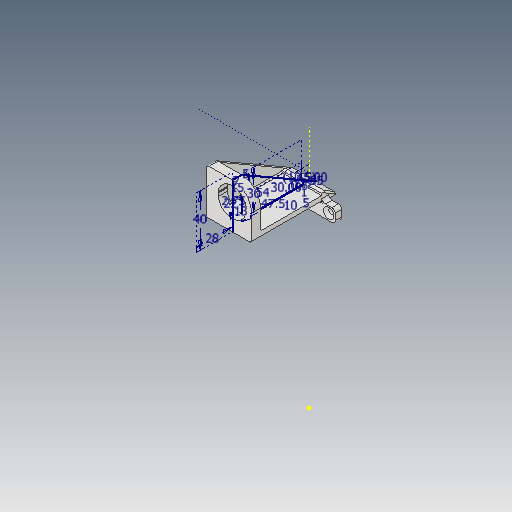
# Autodesk Inventor part: Mount_Killswitch
Saved by Autodesk Inventor 2018.2 (Build 222227000, 227)
## iProperties
Created: 2018-02-23
Part Number: Mount_Killswitch
Material: ABS Plastic
Document SubType Name: Modeling
Designer: NicK Foo
Density: 1.06 g/cm^3
Appearance: Smooth - White
Author: NicK Foo
Autodesk Inventor part; units mm, degrees
ref_plane "YZ Plane" through (0, 0, 0) normal (1, 0, 0) x (0, 1, 0)
ref_plane "XZ Plane" through (0, 0, 0) normal (0, 1, 0) x (-1, 0, 0)
ref_plane "XY Plane" through (0, 0, 0) normal (0, 0, 1) x (1, 0, 0)
sketch "Sketch1" plane through (0, 0, 0) normal (0, 0, 1) x (1, 0, 0)
  circle A0 centre (20, 143.6138) radius 1.7 projected
  circle A1 centre (-20, 143.6138) radius 1.7 projected
  line L0 (37.5, 138.6138) -> (-37.5, 138.6138) projected
  line L1 (20, 138.6138) -> (20, 148.6138)
  circle A2 centre (0, 168.6138) radius 20
  line L2 (25, 138.6138) -> (-25, 138.6138)
  line L3 (-25, 138.6138) -> (-25, 148.6138)
  line L4 (-25, 148.6138) -> (25, 148.6138)
  line L5 (25, 148.6138) -> (25, 138.6138)
  point P0 (0, 0)
  dimension "d0" = 40
  dimension "d1" = 20
  dimension "d41" = 5
  dimension "d42" = 5
  constraints: 10 end point, 4 point on line, 2 parallel, 1 centre point, 1 coincident, 1 midpoint, 1 perpendicular, 1 vertical, 1 vertical alignment
  measures "d0" diameter of A2
  measures "d1" horizontal distance of L1.end A2.centre
  measures "d41" distance from line of L5 A0.centre
  measures "d42" distance from line of L3 A1.centre
sketch "Sketch2" plane through (0, 0, 0) normal (1, 0, 0) x (0, 1, 0)
  line L0 (188.6138, 0) -> (148.6138, 0) construction
  line L1 (157.6138, 60) -> (179.6138, 60) construction
  line L2 (179.6138, 60) -> (179.6138, 47) construction
  line L3 (179.6138, 47) -> (157.6138, 47)
  line L4 (157.6138, 47) -> (157.6138, 60) construction
  line L5 (168.6138, 60) -> (168.6138, 6) construction
  line L6 (148.6138, 60) -> (188.6138, 60) construction
  line L7 (188.6138, 60) -> (188.6138, 88) construction
  line L8 (188.6138, 88) -> (148.6138, 88) construction
  line L9 (148.6138, 88) -> (148.6138, 60) construction
  line L10 (153.6138, 47) -> (153.6138, 6)
  line L11 (153.6138, 6) -> (183.6138, 6) construction
  line L12 (183.6138, 6) -> (183.6138, 47) construction
  line L13 (183.6138, 47) -> (153.6138, 47) construction
  line L14 (138.6138, 0) -> (148.6138, 0) projected
  line L15 (138.6138, 0) -> (138.6138, 5)
  line L16 (138.6138, 5) -> (148.6138, 5)
  line L17 (153.1138, 5) -> (153.1138, 0) construction
  line L18 (153.1138, 0) -> (138.6138, 0) construction
  line L19 (148.6138, 60) -> (148.6138, 5)
  line L20 (148.6138, -5) -> (150.2837, -5)
  line L21 (153.1138, -5) -> (153.1138, 5.5) construction
  line L22 (153.1138, 60) -> (148.6138, 60)
  line L23 (153.1138, -5) -> (246.1138, 88) construction
  line L24 (148.6138, 60) -> (183.6138, 60)
  line L25 (183.6138, 60) -> (183.6138, 53)
  line L26 (183.6138, 53) -> (153.1138, 53)
  line L27 (148.6138, 53) -> (148.6138, 60)
  line L28 (183.6138, 52.0495) -> (183.6138, 47.0495) construction
  line L29 (183.6138, 47.0495) -> (153.6138, 47.0495) construction
  line L30 (153.6138, 47.0495) -> (153.6138, 52.0495) construction
  line L31 (153.6138, 52.0495) -> (183.6138, 52.0495) construction
  line L32 (169.9888, 47) -> (169.9888, 60) construction
  line L33 (167.2388, 60) -> (167.2388, 47) construction
  line L34 (153.1138, 5.5) -> (154.6138, 5.5)
  line L35 (154.6138, 5.5) -> (154.6138, 2.5)
  line L36 (153.1138, 5.5) -> (153.1138, 53)
  line L37 (148.6138, 5) -> (153.1138, 5) construction
  line L38 (148.6138, 5) -> (148.6138, 0) construction
  line L39 (138.6138, 0) -> (148.6138, 0) construction
  line L40 (148.6138, 0) -> (148.6138, -5)
  line L41 (150.2837, -5) -> (153.1138, -5) construction
  line L42 (153.1138, 53) -> (153.1138, 60) construction
  line L43 (153.1138, 53) -> (148.6138, 53) construction
  line L44 (183.6138, 53) -> (183.6138, 52.7295)
  line L45 (150.2837, -5) -> (183.6138, 52.7295)
  line L46 (148.6138, 0) -> (138.6138, 0)
  point P0 (0, 0)
  point P1 (168.6138, 47)
  point P2 (164.1138, 6)
  dimension "d2" = 54
  dimension "d3" = 22
  dimension "d4" = 13
  dimension "d5" = 28
  dimension "d6" = 40
  dimension "d7" = 30
  dimension "d8" = 5
  dimension "d9" = 4.5
  dimension "d10" = 0.5
  dimension "d11" = 5
  dimension "d13" = 45
  dimension "d14" = 15
  dimension "d15" = 7
  dimension "d16" = 5
  dimension "d17" = 2.75
  dimension "d18" = 10.5
  dimension "d19" = 10
  dimension "d20" = 1
  dimension "d21" = 1.5
  dimension "d22" = 3
  dimension "d23" = 47.5
  dimension "d25" = 30
  constraints: 90 end point, 25 parallel, 18 perpendicular, 9 point on line, 8 vertical, 7 collinear, 5 midpoint, 3 horizontal, 2 other
  measures "d2" distance of L5.start L5.end
  measures "d3" distance of L1.start L1.end
  measures "d4" distance of L3.end L1.start
  measures "d5" distance of L8.end L6.start
  measures "d6" distance of L7.end L8.end
  measures "d7" distance of L12.end L10.start
  measures "d8" distance between parallel lines of L18 L20
  measures "d9" distance of L20.start L21.start
  measures "d10" distance between parallel lines of L10 L17
  measures "d11" distance of L14.start L15.end
  measures "d13" angle of L21 L23
  measures "d14" distance between parallel lines of L25 L5
  measures "d15" distance of L24.end L25.end
  measures "d16" distance of L28.start L28.end
  measures "d17" distance between parallel lines of L32 L33
  measures "d18" distance of L10.end point (164.114, 6)
  measures "d19" distance between parallel lines of L15 L19
  measures "d20" distance between parallel lines of L16 L11
  measures "d21" distance of L21.end L34.end
  measures "d22" distance of L34.end L35.end
  measures "d23" distance between parallel lines of L26 L34
  measures "d25" angle of L36 L45
extrude "Extrusion1" add sketch "Sketch2" along normal mid plane 30 contours L15 L16 L19 L22 L24 L25 L26 L36 L34 L35 L45 L20 L40 L14
extrude "Extrusion2" add sketch "Sketch2" against normal blind 20
extrude "Extrusion3" cut sketch "Sketch2" against normal blind 16 contours L35 L34 L36 L26 L44 L45
fillet "Fillet1" radius 15 1 edges at (15, 183.6138, 56.5)
sketch "Sketch3" plane through (-20, 148.6138, 60) normal (0, 0, 1) x (1, 0, 0)
  circle A0 centre (20, 20) radius 20 construction
  circle A1 centre (20, 20) radius 11.05
  line L0 (30.9641, 18.625) -> (30.25, 18.625)
  line L1 (30.9641, 21.375) -> (30.25, 21.375)
  line L2 (30.25, 18.625) -> (30.25, 21.375)
  line L3 (9.75, 18.625) -> (9.75, 21.375)
  line L4 (20, 18.625) -> (20, 21.375) construction
  line L5 (9.75, 18.625) -> (9.0359, 18.625)
  line L6 (30.25, 18.625) -> (9.75, 18.625) construction
  line L7 (30.25, 21.375) -> (9.75, 21.375) construction
  line L8 (9.75, 21.375) -> (9.0359, 21.375)
  point P0 (20, -148.6138)
  dimension "d33" = 22.1
  dimension "d34" = 20.5
  constraints: 18 end point, 6 horizontal, 4 point on circle, 3 point on line, 2 midpoint, 2 vertical, 1 centre point, 1 coincident, 1 parallel, 1 other
  measures "d33" diameter of A1
  measures "d34" distance between parallel lines of L3 L2
extrude "Extrusion4" cut sketch "Sketch3" against normal blind 10 contours L1 L2 L0 A1 L5 L3 L8
fillet "Fillet2" radius 0.1 4 edges at (-10.9641, 169.9888, 56.5) (-10.9641, 167.2388, 56.5) (10.9641, 167.2388, 56.5) (10.9641, 169.9888, 56.5)
fillet "Fillet2" radius 0.25 4 edges at (-10.25, 169.9888, 56.5) (-10.25, 167.2388, 56.5) (10.25, 167.2388, 56.5) (10.25, 169.9888, 56.5)
fillet "Fillet3" radius 1 3 edges at (-16, 168.3638, 53) (-0.5, 153.1138, 53) (-16, 153.1138, 29.25)
fillet "Fillet4" radius 2 2 edges at (-20, 183.6138, 56.3647) (-20, 166.9487, 23.8647)
extrude "Extrusion5" add sketch "Sketch1" along normal blind 5 contours A0 L1 | A0 L1 L4 L5 L0 | L1 A0 | A0 L1 L0 L3 L4 | A1
fillet "Fillet5" radius 2.5 6 edges at (-20, 148.6138, 2.5) (-25, 148.6138, 2.5) (-25, 138.6138, 2.5) (15, 148.6138, 2.5) (25, 148.6138, 2.5) (25, 138.6138, 2.5)
fillet "Fillet5" radius 1 4 edges at (-20, 148.6138, 32.5) (15, 148.6138, 32.5) (-2.5, 148.6138, 5) (15, 152.4487, -1.25)
sketch "Sketch4" plane through (-22.5, 138.6138, 5) normal (0, 0, 1) x (1, 0, 0)
  point P0 (22.5, -138.6138)
  point P1 (42.5, 5)
  point P2 (2.5, 5)
hole "Hole1" at (20, 143.6138, 5) at (-20, 143.6138, 5) direction (0, 0, -1) diameter 4 end through all countersink diameter 8 countersink angle 90
equation "\"d42\" = d41"
body "Solid1"
